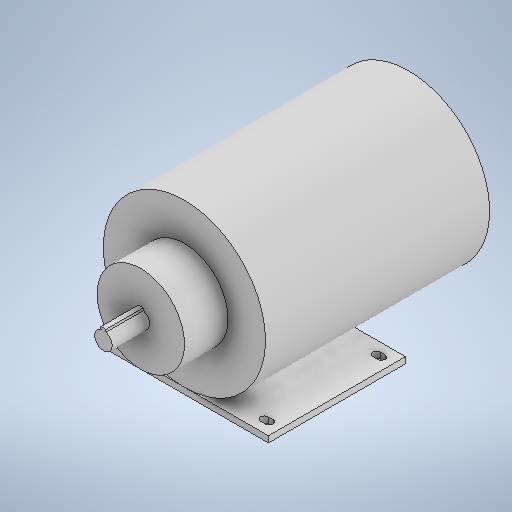
# Autodesk Inventor part: MotorV1
Saved by Autodesk Inventor 2025.1 (Build 291241000, 241)
## iProperties
Created: 2025-10-12
Part Number: MotorV1
Material: Generic
Document SubType Name: Modeling
Designer: jonas
Density: 1 g/cm^3
Appearance: Default
Author: jonas
Autodesk Inventor part; units mm, degrees
ref_plane "YZ Plane" through (0, 0, 0) normal (1, 0, 0) x (0, 1, 0)
ref_plane "XZ Plane" through (0, 0, 0) normal (0, 1, 0) x (-1, 0, 0)
ref_plane "XY Plane" through (0, 0, 0) normal (0, 0, 1) x (1, 0, 0)
sketch "Sketch1" plane through (0, 0, 0) normal (0, 1, 0) x (-1, 0, 0)
  line L0 (-70.0685, 0) -> (70.0685, 0) construction
  line L1 (0, -20.6438) -> (0, 20.6438) construction
  line L2 (67.5, -55) -> (-67.5, -55)
  line L3 (-67.5, -55) -> (-67.5, 55)
  line L4 (-67.5, 55) -> (67.5, 55)
  line L5 (67.5, 55) -> (67.5, -55)
  point P0 (0, 0)
  point P1 (0, 0)
  dimension "d0" = 110
  dimension "d1" = 135
  constraints: 12 end point, 2 horizontal, 2 midpoint, 2 parallel, 1 coincident, 1 perpendicular, 1 vertical, 2 other
  measures "d0" distance between parallel lines of L4 L2
  measures "d1" distance between parallel lines of L3 L5
extrude "Extrusion1" add sketch "Sketch1" along normal blind 5
sketch "Sketch2" plane through (0, 0, 0) normal (0, -1, 0) x (1, 0, 0)
  line L0 (-161.783, 0) -> (161.783, 0) construction
  line L1 (0, 8.6003) -> (0, -8.6003) construction
  line L2 (-58.2, 45) -> (-54.3, 45) construction
  line L3 (-58.2, 48.05) -> (-54.3, 48.05)
  line L4 (-54.3, 41.95) -> (-58.2, 41.95)
  arc A0 (-58.2, 48.05) -> (-58.2, 41.95) centre (-58.2, 45) ccw
  arc A1 (-54.3, 41.95) -> (-54.3, 48.05) centre (-54.3, 45) ccw
  line L5 (58.2, 45) -> (54.3, 45) construction
  line L6 (58.2, 48.05) -> (54.3, 48.05)
  line L7 (54.3, 41.95) -> (58.2, 41.95)
  arc A2 (58.2, 41.95) -> (58.2, 48.05) centre (58.2, 45) ccw
  arc A3 (54.3, 48.05) -> (54.3, 41.95) centre (54.3, 45) ccw
  line L8 (58.2, -45) -> (54.3, -45) construction
  line L9 (58.2, -41.95) -> (54.3, -41.95)
  line L10 (54.3, -48.05) -> (58.2, -48.05)
  arc A4 (58.2, -48.05) -> (58.2, -41.95) centre (58.2, -45) ccw
  arc A5 (54.3, -41.95) -> (54.3, -48.05) centre (54.3, -45) ccw
  line L11 (-58.2, -45) -> (-54.3, -45) construction
  line L12 (-58.2, -48.05) -> (-54.3, -48.05)
  line L13 (-54.3, -41.95) -> (-58.2, -41.95)
  arc A6 (-58.2, -41.95) -> (-58.2, -48.05) centre (-58.2, -45) ccw
  arc A7 (-54.3, -48.05) -> (-54.3, -41.95) centre (-54.3, -45) ccw
  point P0 (0, 0)
  point P1 (-56.25, 45)
  point P2 (56.25, 45)
  point P3 (56.25, -45)
  point P4 (-56.25, -45)
  point P5 (0, 0)
  point P6 (-61.25, 45)
  point P7 (-51.25, 45)
  dimension "d4" = 112.5
  dimension "d5" = 90
  dimension "d7" = 6.1
  dimension "d8" = 10
  constraints: 36 end point, 18 point on circle, 16 tangent, 8 centre point, 6 midpoint, 5 parallel, 3 equal length, 3 equal radius, 3 horizontal, 2 horizontal alignment, 2 symmetric about line, 2 vertical alignment, 1 coincident, 1 point on line, 1 vertical
  measures "d4" distance of point (56.25, 45) point (-56.25, 45)
  measures "d5" distance of point (-56.25, -45) point (-56.25, 45)
  measures "d7" distance between parallel lines of L4 L3
  measures "d8" distance of point (-51.25, 45) point (-61.25, 45)
extrude "Extrusion2" cut sketch "Sketch2" against normal through all
sketch "Sketch3" plane through (0, 0, 0) normal (0, -1, 0) x (1, 0, 0)
  line L0 (-38.6076, 0) -> (38.6076, 0) construction
  line L1 (0, -3.4177) -> (0, 3.4177) construction
  line L2 (10, -10) -> (-10, -10)
  line L3 (-10, -10) -> (-10, 10)
  line L4 (-10, 10) -> (10, 10)
  line L5 (10, 10) -> (10, -10)
  point P0 (0, 0)
  point P1 (0, 0)
  dimension "d11" = 20
  dimension "d12" = 20
  constraints: 12 end point, 2 horizontal, 2 midpoint, 2 parallel, 1 coincident, 1 perpendicular, 1 vertical, 2 other
  measures "d11" distance of L2.start L2.end
  measures "d12" distance between parallel lines of L4 L2
extrude "Extrusion3" add sketch "Sketch3" against normal blind 70
sketch "Sketch4" plane through (-10, 5, 10) normal (0, 0, 1) x (1, 0, 0)
  line L0 (20, 65) -> (0, 65) projected
  circle A0 centre (10, 65) radius 65
  point P0 (10, -5)
  dimension "d15" = 130
  constraints: 1 centre point, 1 midpoint
  measures "d15" diameter of A0
extrude "Extrusion4" add sketch "Sketch4" along normal up to surface (45 mm away)
sketch "Sketch5" plane through (0, 70, 55) normal (0, 0, 1) x (1, 0, 0)
  line L0 (10, 0) -> (-10, 0) projected
  circle A0 centre (0, 0) radius 35
  point P0 (0, -70)
  dimension "d18" = 70
  constraints: 1 centre point, 1 midpoint
  measures "d18" diameter of A0
extrude "Extrusion5" add sketch "Sketch5" along normal blind 35
sketch "Sketch6" plane through (0, 70, 90) normal (0, 0, 1) x (1, 0, 0)
  arc A0 (-2, 6.7082) -> (2, 6.7082) centre (0, 0) ccw
  circle A1 centre (0, 0) radius 35 projected
  line L0 (-2, 8.7082) -> (2, 8.7082)
  line L1 (2, 8.7082) -> (2, 6.7082)
  line L2 (-2, 6.7082) -> (-2, 8.7082)
  point P0 (0, -70)
  dimension "d21" = 14
  dimension "d23" = 2
  dimension "d26" = 4
  dimension "d27" = 2
  constraints: 6 end point, 2 point on circle, 1 centre point, 1 concentric, 1 horizontal, 1 parallel, 1 perpendicular
  measures "d21" diameter of A0
  measures "d23" distance from line of L1 A0.centre
  measures "d26" distance of L0.end L0.start
  measures "d27" distance of L1.end L0.end
extrude "Extrusion6" add sketch "Sketch6" along normal blind 30 contours L2 L0 L1 A0
sketch "Sketch8" plane through (-10, 5, 10) normal (0, 0, -1) x (-1, 0, 0)
  arc A0 (-12, 71.7082) -> (-8, 71.7082) centre (-10, 65) ccw projected
  circle A1 centre (-10, 65) radius 65
  arc A2 (0, 0.7738) -> (-20, 0.7738) centre (-10, 65) ccw projected
  point P0 (-10, -5)
  constraints: 1 centre point, 1 coincident, 1 concentric
extrude "Extrusion7" add sketch "Sketch8" along normal blind 135
body "Solid1"
